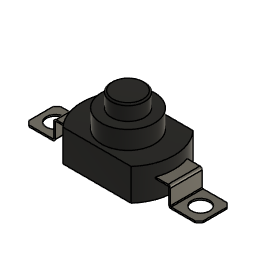
button (Autodesk Fusion 360 design; units mm, degrees)
Autodesk Fusion 360 part; units mm, degrees
sketch "Sketch1" plane through (0, 0, 0) normal (0, 0, 1) x (1, 0, 0)
  line L0 (0, 0) -> (9, 0)
  line L1 (9, 0) -> (9, 8.2)
  line L2 (9, 8.2) -> (0, 8.2)
  line L3 (0, 8.2) -> (0, 0)
  line L4 (4.5, 8.2) -> (4.5, 0) construction
  circle A0 centre (4.5, 4.1) radius 6.0877
  dimension "d1" = 9
  dimension "d2" = 8.2
  dimension "d3" = 12.1754
  constraint horizontal L0
  constraint vertical L1
  constraint horizontal L2
  constraint vertical L3
  constraint coincident L0.start L3.end
  constraint midpoint L2 L4.start
  constraint midpoint L0 L4.end
  constraint midpoint L4 A0.centre
  constraint coincident L1.end A0
  measures "d1" distance of L0.start L0.end
  measures "d2" distance of L0.start L2.end
  measures "d3" diameter of A0
extrude "Extrude1" add sketch "Sketch1" along normal blind 4.2 contours L0 L1 L2 L3 | L3 A0 | L1 A0
sketch "Sketch2" plane through (0, 0, 4.2) normal (0, 0, 1) x (-1, 0, 0)
  arc A0 (-9, 0) -> (-9, -8.2) centre (-4.5, -4.1) ccw
  line L0 (-9, -8.2) -> (0, -8.2)
  arc A1 (0, -8.2) -> (0, 0) centre (-4.5, -4.1) ccw
  line L1 (0, 0) -> (-9, 0)
  circle A2 centre (-4.5, -4.1) radius 3.5
  dimension "d6" = 7
  constraint concentric A0 A2
  measures "d6" diameter of A2
extrude "Extrude2" add sketch "Sketch2" along normal blind 2.4 contours A2
sketch "Sketch3" plane through (0, 0, 6.6) normal (0, 0, 1) x (-1, 0, 0)
  circle A0 centre (-4.5, -4.1) radius 3.5
  circle A1 centre (-4.5, -4.1) radius 2.2
  dimension "d9" = 4.4
  constraint concentric A0 A1
  measures "d9" diameter of A1
extrude "Extrude3" add sketch "Sketch3" along normal blind 2 contours A1
ref_plane "WorkPlane1" through (4.5, 4.1, 2.1) normal (0, -1, 0) x (1, 0, 0)
sketch "Sketch4" plane through (0, 4.1, 0) normal (0, -1, 0) x (-1, 0, 0)
  line L0 (0, -4.2) -> (-9, -4.2)
  line L1 (0, 0) -> (0, -4.2)
  line L2 (0, 0) -> (-9, 0)
  line L3 (-9, 0) -> (-9, -4.2)
  line L4 (-4.5, -4.2) -> (-4.5, 0) construction
  line L5 (-4.5, -2.6) -> (3.2, -2.6)
  line L6 (3.2, -2.6) -> (3.2, -0.2)
  line L7 (3.2, -0.2) -> (7, -0.2)
  line L8 (7, -0.2) -> (7, 0)
  line L9 (7, 0) -> (3, 0)
  line L10 (3, 0) -> (3, -2.4)
  line L11 (3, -2.4) -> (-4.5, -2.4)
  line L12 (-4.5, -2.4) -> (-4.5, -2.6)
  line L13 (3, -2.4) -> (3.2, -2.4) construction
  dimension "d12" = 0.2
  dimension "d13" = 11.5
  dimension "d14" = 3
  dimension "d15" = 2.6
  constraint midpoint L0 L4.start
  constraint midpoint L2 L4.end
  constraint coincident L4 L5.start
  constraint perpendicular L4 L5
  constraint perpendicular L5 L6
  constraint perpendicular L4 L7
  constraint perpendicular L7 L8
  constraint perpendicular L4 L9
  constraint perpendicular L7 L10
  constraint coincident L4 L11.end
  constraint perpendicular L4 L11
  constraint equal L6 L10
  constraint collinear L2 L9
  constraint coincident L6 L13.end
  constraint perpendicular L6 L13
  constraint equal L8 L13
  measures "d12" distance of L7.end L8.end
  measures "d13" distance of L4.end L8
  measures "d14" distance of L1 L10
  measures "d15" distance of L2 L5
extrude "Extrude4" add sketch "Sketch4" along normal mid plane 4.2 contours L1 L5 L6 L7 L8 L9 L10 L11
sketch "Sketch5" plane through (0, 0, 0.2) normal (0, 0, 1) x (-1, 0, 0)
  line L0 (7, -6.2) -> (7, -2)
  line L1 (7, -2) -> (3.2, -2)
  line L2 (3.2, -2) -> (3.2, -6.2)
  line L3 (3.2, -6.2) -> (7, -6.2)
  line L4 (7, -6.2) -> (3.2, -2) construction
  circle A0 centre (5.1, -4.1) radius 1.2
  dimension "d18" = 2.4
  constraint coincident L0.start L3.end
  constraint coincident L1.end L2.start
  constraint midpoint L4 A0.centre
  measures "d18" diameter of A0
extrude "Extrude5" cut sketch "Sketch5" against normal blind 0.2 contours A0
chamfer "Chamfer1" distance 0.5 angle 45 2 edges at (-7, 6.2, 0.1) (-7, 2, 0.1)
fillet "Fillet1" radius 0.1 2 edges at (-3.2, 4.1, 0.2) (-3, 4.1, 2.4)
fillet "Fillet2" radius 0.3 2 edges at (-3.2, 4.1, 2.6) (-3, 4.1, 0)
fillet "Fillet3" radius 0.2 1 edges at (6.5511, 4.8956, 8.6)
pattern_circular "C-Pattern1" count 2 over 360 about axis through (4.5, 4.1, 0) along (0, 0, 1) of "Extrude4", "Extrude5", "Chamfer1", "Fillet1", "Fillet2"
sketch "Sketch6" plane through (0, 0, 0) normal (0, 0, 1) x (1, 0, 0)
move_body "Align1" bodies 1 to x (1, 0, 0) y (0, 1, 0) z (0, 0, 1) at (-4.5, -4.1, 0)
move_body "Move1" bodies 1 to x (1, 0, 0) y (0, 1, 0) z (0, 0, 1) at (0, 0, -2.1)
equation "d13 = ( 23 / 2 ) * 1 mm"
